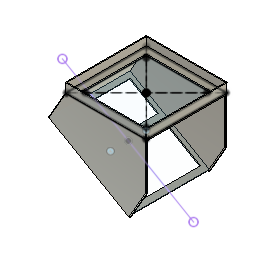
PanaThermoMount_2 (Autodesk Fusion 360 design; units mm, degrees)
part number: 2025-11-09-18-26-20-325
Autodesk Fusion 360 part; units mm, degrees
sketch "BasePlate" plane through (0, 0, 0) normal (0, 0, 1) x (1, 0, 0)
  line L0 (61.5, 62.5) -> (-61.5, 62.5)
  line L1 (-62.5, 61.5) -> (-62.5, -61.5)
  line L2 (-61.5, -62.5) -> (61.5, -62.5)
  line L3 (62.5, -61.5) -> (62.5, 61.5)
  line L4 (62.5, 62.5) -> (-62.5, -62.5) construction
  line L5 (-62.5, 62.5) -> (62.5, -62.5) construction
  line L6 (61, 61) -> (-61, 61)
  line L7 (-61, 61) -> (-61, -61)
  line L8 (-61, -61) -> (61, -61)
  line L9 (61, -61) -> (61, 61)
  line L10 (61, 61) -> (-61, -61) construction
  line L11 (-61, 61) -> (61, -61) construction
  arc A0 (-61.5, 62.5) -> (-62.5, 61.5) centre (-61.5, 61.5) ccw
  arc A1 (62.5, 61.5) -> (61.5, 62.5) centre (61.5, 61.5) ccw
  arc A2 (61.5, -62.5) -> (62.5, -61.5) centre (61.5, -61.5) ccw
  arc A3 (-62.5, -61.5) -> (-61.5, -62.5) centre (-61.5, -61.5) ccw
  line L12 (47, 50) -> (-47, 50)
  line L13 (-50, 47) -> (-50, -47)
  line L14 (-47, -50) -> (47, -50)
  line L15 (50, -47) -> (50, 47)
  line L16 (50, 50) -> (-50, -50) construction
  line L17 (-50, 50) -> (50, -50) construction
  arc A4 (-47, 50) -> (-50, 47) centre (-47, 47) ccw
  arc A5 (50, 47) -> (47, 50) centre (47, 47) ccw
  arc A6 (47, -50) -> (50, -47) centre (47, -47) ccw
  arc A7 (-50, -47) -> (-47, -50) centre (-47, -47) ccw
  dimension "d1" = 125
  dimension "d2" = 125
  dimension "d3" = 122
  dimension "d4" = 122
  dimension "d5" = 1
  dimension "d6" = 100
  dimension "d7" = 100
  dimension "d8" = 3
  constraint horizontal L0
  constraint perpendicular L0 L1
  constraint parallel L0 L2
  constraint parallel L1 L3
  constraint coincident L4 origin
  constraint coincident L5 origin
  constraint horizontal L6
  constraint perpendicular L6 L7
  constraint parallel L6 L8
  constraint parallel L7 L9
  constraint coincident L10 origin
  constraint coincident L11 origin
  constraint coincident L5.start L0
  constraint coincident L5.start L1
  constraint tangent L0 A0
  constraint tangent L1 A0
  constraint coincident L4.start L0
  constraint coincident L4.start L3
  constraint tangent L0 A1
  constraint tangent L3 A1
  constraint equal A0 A1
  constraint coincident L5.end L2
  constraint coincident L5.end L3
  constraint tangent L2 A2
  constraint tangent L3 A2
  constraint equal A0 A2
  constraint coincident L4.end L1
  constraint coincident L4.end L2
  constraint tangent L1 A3
  constraint tangent L2 A3
  constraint equal A0 A3
  constraint horizontal L12
  constraint perpendicular L12 L13
  constraint parallel L12 L14
  constraint parallel L13 L15
  constraint coincident L16 origin
  constraint coincident L17 origin
  constraint coincident L17.start L12
  constraint coincident L17.start L13
  constraint tangent L12 A4
  constraint tangent L13 A4
  constraint coincident L16.start L15
  constraint coincident L16.start L12
  constraint tangent L15 A5
  constraint tangent L12 A5
  constraint equal A4 A5
  constraint coincident L17.end L15
  constraint coincident L17.end L14
  constraint tangent L15 A6
  constraint tangent L14 A6
  constraint equal A4 A6
  constraint coincident L16.end L13
  constraint coincident L16.end L14
  constraint tangent L13 A7
  constraint tangent L14 A7
  constraint equal A4 A7
  measures "d1" distance of L4.end L5.end
  measures "d2" distance of L5.start L4.end
  measures "d3" distance of L7.end L8.end
  measures "d4" distance of L6.end L7.end
  measures "d5" radius of A0
  measures "d6" distance of L16.end L17.end
  measures "d7" distance of L17.start L16.end
  measures "d8" radius of A4
extrude "Extrude1" add sketch "BasePlate" along normal blind 14 contours L0 L1 L2 L3 A0 A1 A2 A3 makes body 1
extrude "Extrude2" add sketch "BasePlate" along normal blind 2 contours L6 L7 L8 L9 bodies 1
extrude "Extrude3" add sketch "BasePlate" against normal blind 100 contours L0 L1 L2 L3 A0 A1 A2 A3 bodies 1
ref_plane "WorkPlane1" through (-62.5, 0, 0) normal (0.5, 0, 0.866025) x (0, -1, 0)
split "Split1" by plane through (-62.5, 0, 0) normal (0.5, 0, 0.866025) bodies 1 makes body 2 at (62.5, -20.5, -43.4459)
delete_body "RemoveBody1" bodies 1
extrude "Extrude4" add 1 faces at (62, -20.3333, -71.8801) along direction (-0.5, 0, -0.866025) blind 50 on bodies 2 bodies 2
sketch "BottomCutter" plane through (62.5, 0, 0) normal (1, 0, 0) x (0, 1, 0)
  line L0 (-61.5, -72.1688) -> (61.5, -72.1688)
  line L1 (61.5, -72.1688) -> (61.5, 14)
  line L2 (61.5, 14) -> (-61.5, 14)
  line L3 (-61.5, 14) -> (-61.5, -72.1688)
  line L4 (-60.0198, -72.1688) -> (60, -72.1688)
  line L5 (60, -72.1688) -> (60, -2)
  line L6 (60, -2) -> (-60.0198, -2)
  line L7 (-60.0198, -2) -> (-60.0198, -72.1688)
  line L8 (60, -142.3376) -> (-60.0198, -142.3376)
  line L9 (-60.0198, -142.3376) -> (-60.0198, -72.1688)
  line L10 (60, -72.1688) -> (60, -142.3376)
  constraint horizontal L4
  constraint vertical L5
  constraint horizontal L6
  constraint vertical L7
  constraint coincident L0 L4.start
  constraint symmetric L7.end L4 L9.end
  constraint symmetric L5.start L4 L10.start
  constraint symmetric L5.end L4 L8.start
  constraint symmetric L6.end L4 L8.end
extrude "Extrude6" cut sketch "BottomCutter" against normal blind 30 contours L0 L4 L5 L6 L7 | L0 L4 L8 L9 L10 bodies 2
sketch "BottomCutter2" plane through (-40.625, 0, -70.3646) normal (-0.5, 0, -0.866025) x (0, -1, 0)
  line L0 (60.0198, -88.4789) -> (60.0198, -90.211)
  line L1 (60.0198, -90.211) -> (61.5, -90.211)
  ellipse E0 centre (61.5, -89.0563) end of major axis (61.5, -90.211) minor radius 1 (61.5, -90.211) -> (62.5, -89.0563) ccw
  line L2 (62.5, -89.0563) -> (62.5, 52.9719)
  ellipse E1 centre (61.5, 52.9719) end of major axis (61.5, 54.1266) minor radius 1 (62.5, 52.9719) -> (61.5, 54.1266) ccw
  line L3 (61.5, 54.1266) -> (-61.5, 54.1266)
  ellipse E2 centre (-61.5, 52.9719) end of major axis (-61.5, 54.1266) minor radius 1 (-61.5, 54.1266) -> (-62.5, 52.9719) ccw
  line L4 (-62.5, 52.9719) -> (-62.5, -89.0563)
  ellipse E3 centre (-61.5, -89.0563) end of major axis (-61.5, -90.211) minor radius 1 (-62.5, -89.0563) -> (-61.5, -90.211) ccw
  line L5 (-61.5, -90.211) -> (-60, -90.211)
  line L6 (-60, -90.211) -> (-60, -88.4789)
  line L7 (-60, -88.4789) -> (-61, -88.4789)
  line L8 (-61, -88.4789) -> (-61, 52.3945)
  line L9 (-61, 52.3945) -> (61, 52.3945)
  line L10 (61, 52.3945) -> (61, -88.4789)
  line L11 (61, -88.4789) -> (60.0198, -88.4789)
  line L12 (-61, 52.3945) -> (61, 52.3945)
  line L13 (61, 52.3945) -> (61, -88.4789)
  line L14 (61, -88.4789) -> (-61, -88.4789)
  line L15 (-61, -88.4789) -> (-61, 52.3945)
  constraint horizontal L12
  constraint vertical L13
  constraint horizontal L14
  constraint vertical L15
  constraint coincident L10 L11.start
  constraint coincident L8.end L9.start
extrude "Extrude7" add sketch "BottomCutter2" along normal blind 2 bodies 2
ref_plane "WorkPlane2" through (-13, 0, -51.3124) normal (0, 1, 0) x (-1, 0, 0)
sketch "MountingHoles" plane through (-40.625, 0, -70.3646) normal (0.5, 0, 0.866025) x (0, 1, 0)
  line L0 (60, -88.4789) -> (61, -88.4789)
  line L1 (61, -88.4789) -> (61, 52.3945)
  line L2 (61, 52.3945) -> (-61, 52.3945)
  line L3 (-61, 52.3945) -> (-61, -88.4789)
  line L4 (-61, -88.4789) -> (-60.0198, -88.4789)
  line L5 (-60.0198, -88.4789) -> (60, -88.4789)
  circle A0 centre (-27.5, -15) radius 2.5
  line L6 (0, 102.2122) -> (0, -131.008)
  circle A1 centre (27.5, -15) radius 2.5
  point P0 (0, -15)
  dimension "d29" = 5
  dimension "d30" = 27.5
  constraint symmetric A0 L6 A1
  constraint coincident L6 P0
  measures "d29" diameter of A0
  measures "d30" distance of A0.centre L6
hole "Hole1" at (-27.6346, -27.5, -77.8646) direction (-0.5, 0, -0.866025) diameter 3.4 depth 2 tip angle 180 countersink diameter 6.3 countersink angle 90 bodies 2
hole "Hole2" at (-27.6346, 27.5, -77.8646) direction (-0.5, 0, -0.866025) diameter 3.4 depth 2 tip angle 180 countersink diameter 6.3 countersink angle 90 bodies 2
sketch "WallSideCutter" plane through (-41.625, 0, -72.0966) normal (-0.5, 0, -0.866025) x (0, -1, 0)
  circle A0 centre (-27.5, -15) radius 1.7
  circle A1 centre (27.5, -15) radius 1.7
  line L0 (60.0198, -88.4789) -> (60.0198, -90.211)
  line L1 (60.0198, -90.211) -> (61.5, -90.211)
  ellipse E0 centre (61.5, -89.0563) end of major axis (61.5, -90.211) minor radius 1 (61.5, -90.211) -> (62.5, -89.0563) ccw
  line L2 (62.5, -89.0563) -> (62.5, 52.9719)
  ellipse E1 centre (61.5, 52.9719) end of major axis (61.5, 54.1266) minor radius 1 (62.5, 52.9719) -> (61.5, 54.1266) ccw
  line L3 (61.5, 54.1266) -> (-61.5, 54.1266)
  ellipse E2 centre (-61.5, 52.9719) end of major axis (-61.5, 54.1266) minor radius 1 (-61.5, 54.1266) -> (-62.5, 52.9719) ccw
  line L4 (-62.5, 52.9719) -> (-62.5, -89.0563)
  ellipse E3 centre (-61.5, -89.0563) end of major axis (-61.5, -90.211) minor radius 1 (-62.5, -89.0563) -> (-61.5, -90.211) ccw
  line L5 (-61.5, -90.211) -> (-60, -90.211)
  line L6 (-60, -90.211) -> (-60, -88.4789)
  line L7 (-60, -88.4789) -> (60.0198, -88.4789)
  line L8 (-55, 45) -> (55, 45)
  line L9 (55, 45) -> (55, -5)
  line L10 (55, -5) -> (-55, -5)
  line L11 (-55, -5) -> (-55, 45)
  line L12 (-55, -25) -> (55, -25)
  line L13 (55, -25) -> (55, -80)
  line L14 (55, -80) -> (-55, -80)
  line L15 (-55, -80) -> (-55, -25)
  constraint horizontal L8
  constraint vertical L9
  constraint horizontal L10
  constraint vertical L11
  constraint horizontal L12
  constraint vertical L13
  constraint horizontal L14
  constraint vertical L15
extrude "Extrude9" cut sketch "WallSideCutter" against normal blind 2 contours L8 L9 L10 L11 | L12 L13 L14 L15 bodies 2
named bodies: "Holder"
